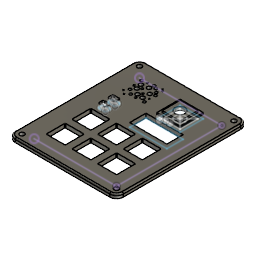
Assembly Macropad (Autodesk Fusion 360 archive; units mm, degrees)
design "Macro Pad top"
part number: 2026-02-01-14-28-44-356
Autodesk Fusion 360 part; units mm, degrees
sketch "Sketch1" plane through (0, 0, 0) normal (0, 0, 1) x (1, 0, 0)
  line L0 (9.1178, 38.3156) -> (22.1178, 38.3156)
  line L1 (9.1178, 24.3156) -> (22.1178, 24.3156)
  line L2 (8.6178, 37.8156) -> (8.6178, 24.8156)
  line L3 (22.6178, 37.8156) -> (22.6178, 24.8156)
  arc A0 (9.1178, 38.3156) -> (8.6178, 37.8156) centre (9.1178, 37.8156) ccw
  arc A1 (22.6178, 37.8156) -> (22.1178, 38.3156) centre (22.1178, 37.8156) ccw
  arc A2 (8.6178, 24.8156) -> (9.1178, 24.3156) centre (9.1178, 24.8156) ccw
  arc A3 (22.1178, 24.3156) -> (22.6178, 24.8156) centre (22.1178, 24.8156) ccw
  line L4 (28.1678, 38.3156) -> (41.1678, 38.3156)
  line L5 (28.1678, 24.3156) -> (41.1678, 24.3156)
  line L6 (27.6678, 37.8156) -> (27.6678, 24.8156)
  line L7 (41.6678, 37.8156) -> (41.6678, 24.8156)
  arc A4 (28.1678, 38.3156) -> (27.6678, 37.8156) centre (28.1678, 37.8156) ccw
  arc A5 (41.6678, 37.8156) -> (41.1678, 38.3156) centre (41.1678, 37.8156) ccw
  arc A6 (27.6678, 24.8156) -> (28.1678, 24.3156) centre (28.1678, 24.8156) ccw
  arc A7 (41.1678, 24.3156) -> (41.6678, 24.8156) centre (41.1678, 24.8156) ccw
  line L8 (47.2178, 38.3156) -> (60.2178, 38.3156)
  line L9 (47.2178, 24.3156) -> (60.2178, 24.3156)
  line L10 (46.7178, 37.8156) -> (46.7178, 24.8156)
  line L11 (60.7178, 37.8156) -> (60.7178, 24.8156)
  arc A8 (47.2178, 38.3156) -> (46.7178, 37.8156) centre (47.2178, 37.8156) ccw
  arc A9 (60.7178, 37.8156) -> (60.2178, 38.3156) centre (60.2178, 37.8156) ccw
  arc A10 (46.7178, 24.8156) -> (47.2178, 24.3156) centre (47.2178, 24.8156) ccw
  arc A11 (60.2178, 24.3156) -> (60.7178, 24.8156) centre (60.2178, 24.8156) ccw
  line L12 (9.1178, 19.2656) -> (22.1178, 19.2656)
  line L13 (9.1178, 5.2656) -> (22.1178, 5.2656)
  line L14 (8.6178, 18.7656) -> (8.6178, 5.7656)
  line L15 (22.6178, 18.7656) -> (22.6178, 5.7656)
  arc A12 (9.1178, 19.2656) -> (8.6178, 18.7656) centre (9.1178, 18.7656) ccw
  arc A13 (22.6178, 18.7656) -> (22.1178, 19.2656) centre (22.1178, 18.7656) ccw
  arc A14 (8.6178, 5.7656) -> (9.1178, 5.2656) centre (9.1178, 5.7656) ccw
  arc A15 (22.1178, 5.2656) -> (22.6178, 5.7656) centre (22.1178, 5.7656) ccw
  line L16 (28.1678, 19.2656) -> (41.1678, 19.2656)
  line L17 (28.1678, 5.2656) -> (41.1678, 5.2656)
  line L18 (27.6678, 18.7656) -> (27.6678, 5.7656)
  line L19 (41.6678, 18.7656) -> (41.6678, 5.7656)
  arc A16 (28.1678, 19.2656) -> (27.6678, 18.7656) centre (28.1678, 18.7656) ccw
  arc A17 (41.6678, 18.7656) -> (41.1678, 19.2656) centre (41.1678, 18.7656) ccw
  arc A18 (27.6678, 5.7656) -> (28.1678, 5.2656) centre (28.1678, 5.7656) ccw
  arc A19 (41.1678, 5.2656) -> (41.6678, 5.7656) centre (41.1678, 5.7656) ccw
  line L20 (47.2178, 19.2656) -> (60.2178, 19.2656)
  line L21 (47.2178, 5.2656) -> (60.2178, 5.2656)
  line L22 (46.7178, 18.7656) -> (46.7178, 5.7656)
  line L23 (60.7178, 18.7656) -> (60.7178, 5.7656)
  arc A20 (47.2178, 19.2656) -> (46.7178, 18.7656) centre (47.2178, 18.7656) ccw
  arc A21 (60.7178, 18.7656) -> (60.2178, 19.2656) centre (60.2178, 18.7656) ccw
  arc A22 (46.7178, 5.7656) -> (47.2178, 5.2656) centre (47.2178, 5.7656) ccw
  arc A23 (60.2178, 5.2656) -> (60.7178, 5.7656) centre (60.2178, 5.7656) ccw
  circle A24 centre (69.6528, -3.6994) radius 1.7
  circle A25 centre (69.6528, 83.3006) radius 1.7
  line L24 (65.1528, 0.8006) -> (65.1528, 78.8006)
  line L25 (74.6528, 88.3006) -> (-5.3472, 88.3006)
  line L26 (4.1528, 78.8006) -> (4.1528, 0.8006)
  circle A26 centre (-0.3472, -3.6994) radius 1.7
  circle A27 centre (69.6528, -3.6994) radius 3
  circle A28 centre (69.6528, 83.3006) radius 3
  line L27 (-5.3472, -8.6994) -> (74.6528, -8.6994)
  circle A29 centre (-0.3472, 83.3006) radius 1.7
  line L28 (-5.3472, 88.3006) -> (-5.3472, -8.6994)
  line L29 (4.1528, 0.8006) -> (65.1528, 0.8006)
  circle A30 centre (-0.3472, 83.3006) radius 3
  line L30 (65.1528, 78.8006) -> (4.1528, 78.8006)
  line L31 (74.6528, -8.6994) -> (74.6528, 88.3006)
  circle A31 centre (-0.3472, -3.6994) radius 3
  line L32 (4.1528, 78.8006) -> (7.6528, 78.8006)
  line L33 (7.6528, 78.8006) -> (25.6528, 78.8006)
  line L34 (25.6528, 78.8006) -> (25.6528, 57.8006)
  line L35 (25.6528, 57.8006) -> (7.6528, 57.8006)
  line L36 (7.6528, 57.8006) -> (7.6528, 78.8006)
  point P0 (4.1528, 0.8006)
  dimension "d1" = 61
  dimension "d2" = 78
  dimension "d3" = 80
  dimension "d4" = 97
  dimension "d5" = 9.5
  dimension "d6" = 9.5
  dimension "d7" = 9.5
  dimension "d8" = 3.4
  dimension "d9" = 3.4
  dimension "d10" = 3.4
  dimension "d11" = 3.4
  dimension "d12" = 5
  dimension "d13" = 5
  dimension "d14" = 5
  dimension "d15" = 5
  dimension "d16" = 5
  dimension "d17" = 5
  dimension "d18" = 5
  dimension "d19" = 5
  dimension "d20" = 6
  dimension "d21" = 6
  dimension "d22" = 6
  dimension "d23" = 6
  dimension "d27" = 13.965
  dimension "d28" = 13.935
  dimension "d29" = 4.465
  dimension "d75" = 3.5
  dimension "d76" = 18
  dimension "d77" = 21
  constraint horizontal L29
  constraint vertical L24
  constraint horizontal L30
  constraint vertical L26
  constraint horizontal L25
  constraint vertical L28
  constraint horizontal L27
  constraint vertical L31
  constraint coincident P0 L26.end
  constraint concentric A26 A31
  constraint concentric A24 A27
  constraint concentric A25 A28
  constraint concentric A29 A30
  constraint perpendicular L26 L32
  constraint horizontal L33
  constraint vertical L34
  constraint horizontal L35
  constraint vertical L36
  measures "d1" distance of P0 L24.start
  measures "d2" distance of L26.start P0
  measures "d3" distance of L25.start L25.end
  measures "d4" distance of L25.start L27.end
  measures "d5" distance of L24 L31
  measures "d6" distance of L26 L28
  measures "d7" distance of L26.start L25
  measures "d8" diameter of A26
  measures "d9" diameter of A24
  measures "d10" diameter of A25
  measures "d11" diameter of A29
  measures "d12" distance of A26.centre L27
  measures "d13" distance of A26.centre L28
  measures "d14" distance of A24.centre L27
  measures "d15" distance of A24.centre L31
  measures "d16" distance of A25.centre L31
  measures "d17" distance of A25.centre L25
  measures "d18" distance of A29.centre L25
  measures "d19" distance of A29.centre L28
  measures "d20" diameter of A31
  measures "d21" diameter of A27
  measures "d22" diameter of A28
  measures "d23" diameter of A30
  measures "d27" distance of L14 L28
  measures "d28" distance of L23 L31
  measures "d29" distance of L17 L29
  measures "d75" distance of L26.start L32.end
  measures "d76" distance of L32.end L33.end
  measures "d77" distance of L32.end L35.end
sketch "Sketch2" plane through (0, 0, 0) normal (0, 0, 1) x (1, 0, 0)
  line L0 (4.1528, 0.8006) -> (65.1528, 0.8006)
  line L1 (59.67, 43.6006) -> (32.17, 43.6006)
  line L2 (32.17, 43.6006) -> (32.17, 55.6006)
  line L3 (32.17, 55.6006) -> (59.67, 55.6006)
  line L4 (59.67, 55.6006) -> (59.67, 43.6006)
  line L5 (8.9, 44.3006) -> (12.5, 44.3006)
  line L6 (13.5, 45.3006) -> (13.5, 47.3006)
  line L7 (12.5, 48.3006) -> (8.9, 48.3006)
  line L8 (7.9, 47.3006) -> (7.9, 45.3006)
  line L9 (8.9, 51.3006) -> (12.5, 51.3006)
  line L10 (13.5, 52.3006) -> (13.5, 54.3006)
  line L11 (12.5, 55.3006) -> (8.9, 55.3006)
  line L12 (7.9, 54.3006) -> (7.9, 52.3006)
  arc A0 (8.9, 55.3006) -> (7.9, 54.3006) centre (8.9, 54.3006) ccw
  arc A1 (13.5, 54.3006) -> (12.5, 55.3006) centre (12.5, 54.3006) ccw
  arc A2 (12.5, 51.3006) -> (13.5, 52.3006) centre (12.5, 52.3006) ccw
  arc A3 (7.9, 52.3006) -> (8.9, 51.3006) centre (8.9, 52.3006) ccw
  arc A4 (8.9, 48.3006) -> (7.9, 47.3006) centre (8.9, 47.3006) ccw
  arc A5 (13.5, 47.3006) -> (12.5, 48.3006) centre (12.5, 47.3006) ccw
  arc A6 (7.9, 45.3006) -> (8.9, 44.3006) centre (8.9, 45.3006) ccw
  arc A7 (12.5, 44.3006) -> (13.5, 45.3006) centre (12.5, 45.3006) ccw
  line L13 (44.7028, 61.0006) -> (38.8028, 61.0006)
  line L14 (38.8028, 61.0006) -> (52.0028, 61.0006)
  line L15 (52.0028, 61.0006) -> (52.0028, 74.2006)
  line L16 (52.0028, 74.2006) -> (38.8028, 74.2006)
  line L17 (38.8028, 74.2006) -> (38.8028, 61.0006)
  line L18 (38.8028, 61.0006) -> (52.0028, 74.2006)
  line L19 (38.8028, 74.2006) -> (52.0028, 61.0006)
  circle A8 centre (45.4028, 67.6006) radius 3.7
  line L20 (65.1528, 0.8006) -> (65.1528, 78.8006)
  line L21 (65.1528, 78.8006) -> (4.1528, 78.8006)
  line L22 (38.8028, 61.0006) -> (41.3028, 61.0006) construction
  line L23 (38.8028, 61.0006) -> (38.8028, 59.0006)
  line L24 (38.8028, 61.0006) -> (36.8028, 61.0006)
  line L25 (36.8, 59) -> (54, 59)
  line L26 (54, 59) -> (54, 76.2)
  line L27 (54, 76.2) -> (36.8, 76.2)
  line L28 (36.8, 76.2) -> (36.8, 59)
  point P0 (13.5, 44.3006)
  point P1 (13.5, 51.3006)
  point P2 (7.9, 55.3006)
  dimension "d32" = 27.5
  dimension "d33" = 12
  dimension "d41" = 1
  dimension "d42" = 1
  dimension "d43" = 1
  dimension "d44" = 1
  dimension "d45" = 1
  dimension "d46" = 1
  dimension "d47" = 1
  dimension "d48" = 1
  dimension "d51" = 5.9
  dimension "d53" = 13.2
  dimension "d54" = 13.2
  dimension "d55" = 7.4
  dimension "d56" = 13.15
  dimension "d57" = 4.6
  dimension "d64" = 2
  dimension "d65" = 2
  dimension "d66" = 17.2
  dimension "d67" = 17.2
  constraint horizontal L1
  constraint vertical L2
  constraint horizontal L3
  constraint vertical L4
  constraint horizontal L5
  constraint vertical L6
  constraint horizontal L7
  constraint vertical L8
  constraint horizontal L9
  constraint vertical L10
  constraint horizontal L11
  constraint vertical L12
  constraint coincident P2 L11
  constraint coincident P2 L12
  constraint tangent L11 A0
  constraint tangent L12 A0
  constraint tangent L11 A1
  constraint tangent L10 A1
  constraint coincident P1 L10
  constraint coincident P1 L9
  constraint tangent L10 A2
  constraint tangent L9 A2
  constraint tangent L12 A3
  constraint tangent L9 A3
  constraint tangent L8 A4
  constraint tangent L7 A4
  constraint tangent L6 A5
  constraint tangent L7 A5
  constraint tangent L5 A6
  constraint tangent L8 A6
  constraint coincident P0 L5
  constraint coincident P0 L6
  constraint tangent L5 A7
  constraint tangent L6 A7
  constraint horizontal L13
  constraint horizontal L14
  constraint vertical L15
  constraint horizontal L16
  constraint vertical L17
  constraint midpoint L19 A8.centre
  constraint horizontal L22
  constraint perpendicular L13 L23
  constraint perpendicular L23 L24
  constraint horizontal L25
  constraint vertical L26
  constraint horizontal L27
  constraint vertical L28
  measures "d32" distance of L1.start L1.end
  measures "d33" distance of L1.start L3.end
  measures "d41" radius of A0
  measures "d42" radius of A1
  measures "d43" radius of A2
  measures "d44" radius of A3
  measures "d45" radius of A4
  measures "d46" radius of A5
  measures "d47" radius of A6
  measures "d48" radius of A7
  measures "d51" distance of L13.start L13.end
  measures "d53" distance of L13.end L14.end
  measures "d54" distance of L13.end L16.end
  measures "d55" diameter of A8
  measures "d56" distance of L15 L20
  measures "d57" distance of L16 L21
  measures "d64" distance of L13.end L23.end
  measures "d65" distance of L13.end L24.end
  measures "d66" distance of L25.start L25.end
  measures "d67" distance of L25.start L27.end
extrude "Extrude1" add sketch "Sketch1" along normal blind 1.5 contours L24 L26 L29 L30 L32 L34 L35 L36 | L30 L33 L34 L35 L36 | L25 L27 L28 L31 | A27 | A28 | A30 | A31 makes body 1
extrude "Extrude2" cut sketch "Sketch2" along normal blind 3 contours L1 L2 L3 L4 | L5 L6 L7 L8 A4 A5 A6 A7 | L9 L10 L11 L12 A0 A1 A2 A3 | L13 L14 L18 L19 A8 | L17 L18 L19 A8 | L15 L18 L19 A8 | L16 L18 L19 A8 | L18 L19 A8 | L18 L19 A8 | L18 L19 A8 | L18 L19 A8 bodies 1
extrude "Extrude3" cut sketch "Sketch2" along normal blind 2.8 contours L25 L26 L27 L28 bodies 1
extrude "Extrude4" add sketch "Sketch2" along normal blind 2.8 contours L25 L26 L27 L28 bodies 1
extrude "Extrude5" add sketch "Sketch2" along normal blind 1.5 from surface at 2.8 separate body contours L13 L14 L18 L19 A8 | L17 L18 L19 A8 | L15 L18 L19 A8 | L16 L18 L19 A8 makes body 2
sketch "Sketch3" plane through (0, 0, 0) normal (0, 0, 1) x (1, 0, 0)
sketch "Sketch4" plane through (0, 0, 0) normal (0, 0, 1) x (1, 0, 0)
  line L0 (7.6137, 57.8503) -> (25.5702, 78.6939)
  circle A0 centre (10.9555, 65.0578) radius 1
  circle A1 centre (12.9762, 68.0439) radius 1.5
  circle A2 centre (17.0107, 73.0161) radius 1.5
  circle A3 centre (12.0039, 72.0507) radius 1.5
  circle A4 centre (14.99, 70.03) radius 0.75
  circle A5 centre (20.0245, 74.9953) radius 1
  circle A6 centre (9.9832, 69.0646) radius 0.75
  circle A7 centre (8.9348, 62.0717) radius 0.5
  circle A8 centre (23.0382, 76.9746) radius 0.5
  circle A9 centre (17.6448, 76.2674) radius 1
  circle A10 centre (13.2878, 75.4618) radius 0.5
  circle A11 centre (9.4884, 75.0399) radius 1
  circle A12 centre (16.9014, 64.6624) radius 1.5
  circle A13 centre (14.2473, 62.222) radius 1
  circle A14 centre (18.3539, 61.8534) radius 0.75
  circle A15 centre (21.008, 64.2938) radius 1.5
  circle A16 centre (11.5931, 59.7816) radius 0.5
  circle A17 centre (21.2218, 69.3883) radius 1.5
  circle A18 centre (18.5676, 66.948) radius 0.75
  circle A19 centre (22.7332, 72.6618) radius 1
  circle A20 centre (24.3434, 70.4966) radius 1
  circle A21 centre (24.1915, 66.0684) radius 0.5
  circle A22 centre (24.3365, 62.2485) radius 1
  circle A23 centre (24.2445, 75.9353) radius 0.5
  dimension "d78" = 2
  dimension "d79" = 3
  dimension "d81" = 3
  dimension "d82" = 3
  dimension "d84" = 1.5
  dimension "d85" = 2
  dimension "d86" = 1.5
  dimension "d87" = 1
  dimension "d88" = 1
  dimension "d89" = 2
  dimension "d90" = 1
  dimension "d91" = 2
  constraint symmetric L0 A0 A13
  constraint symmetric L0 A1 A12
  constraint symmetric L0 A2 A17
  constraint symmetric L0 A3 A15
  constraint symmetric L0 A4 A18
  constraint symmetric L0 A5 A19
  constraint symmetric L0 A6 A14
  constraint symmetric L0 A7 A16
  constraint symmetric L0 A8 A23
  constraint symmetric L0 A9 A20
  constraint symmetric L0 A10 A21
  constraint symmetric L0 A11 A22
  measures "d78" diameter of A0
  measures "d79" diameter of A1
  measures "d81" diameter of A2
  measures "d82" diameter of A3
  measures "d84" diameter of A4
  measures "d85" diameter of A5
  measures "d86" diameter of A6
  measures "d87" diameter of A7
  measures "d88" diameter of A8
  measures "d89" diameter of A9
  measures "d90" diameter of A10
  measures "d91" diameter of A11
extrude "Extrude6" cut sketch "Sketch4" along normal blind 5 bodies 1
extrude "Extrude7" add 1 faces at (70.0078, 39.1389, 1.5) along direction (0, 0, 1) blind 2 on bodies 1 bodies 1
extrude "Extrude8" add sketch "Sketch2" along normal blind 4 separate body contours L25 L26 L27 L28 makes body 3
extrude "Extrude9" cut 1 faces at (70.0078, 39.1389, 3.5) along direction (0, 0, -1) blind 0.5 on bodies 1 bodies 1
extrude "Extrude10" add 1 faces at (39.7726, 67.5126, 4.3) along direction (0, 0, 1) blind 1 on bodies 2 bodies 2
fillet "Fillet1" radius 5 4 edges at (74.6528, 88.3006, 1.5) (74.6528, -8.6994, 1.5) (-5.3472, -8.6994, 1.5) (-5.3472, 88.3006, 1.5) on bodies 1
fillet "Fillet2" radius 1 8 edges at (34.6528, -8.6994, 3) (-3.8827, -7.235, 3) (-5.3472, 39.8006, 3) (-3.8827, 86.8361, 3) (34.6528, 88.3006, 3) (73.1884, 86.8361, 3) (74.6528, 39.8006, 3) (73.1884, -7.235, 3) on bodies 1
equation "d27 = 4.465 mm + 9.5 mm"
